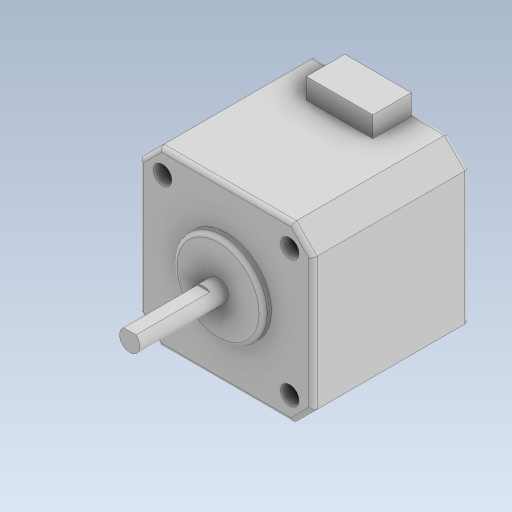
# Autodesk Inventor part: Motor Model
Saved by Autodesk Inventor 2023 (Build 270158000, 158)
## iProperties
Created: 2022-11-09
Part Number: Motor Model
Material: Generic
Document SubType Name: Modeling
Designer: Dave
Density: 1 g/cm^3
Appearance: Default
Author: Dave
Autodesk Inventor part; units mm, degrees
ref_plane "YZ Plane" through (0, 0, 0) normal (1, 0, 0) x (0, 1, 0)
ref_plane "XZ Plane" through (0, 0, 0) normal (0, 1, 0) x (-1, 0, 0)
ref_plane "XY Plane" through (0, 0, 0) normal (0, 0, 1) x (1, 0, 0)
sketch "Sketch1" plane through (0, 0, 0) normal (0, 0, 1) x (1, 0, 0)
  line L0 (5, 0) -> (37.3, 0)
  line L1 (42.3, 5) -> (42.3, 37.3)
  line L2 (37.3, 42.3) -> (5, 42.3)
  line L3 (0, 37.3) -> (0, 5)
  line L4 (5, 42.3) -> (0, 37.3)
  line L5 (42.3, 37.3) -> (37.3, 42.3)
  line L6 (37.3, 0) -> (42.3, 5)
  line L7 (0, 5) -> (5, 0)
  point P0 (0, 0)
  point P1 (42.3, 42.3)
  point P2 (42.3, 0)
  point P3 (0, 42.3)
  dimension "d0" = 42.3
  dimension "d1" = 42.3
  dimension "d2" = 5
  dimension "d3" = 5
  dimension "d4" = 5
  dimension "d5" = 5
  dimension "d6" = 5
  dimension "d7" = 5
  dimension "d8" = 5
  dimension "d9" = 5
  constraints: 16 end point, 8 point on line, 2 parallel, 1 horizontal, 1 perpendicular
  measures "d0" distance of point (0, 42.3) point (42.3, 42.3)
  measures "d1" distance of point (42.3, 42.3) point (42.3, 0)
  measures "d2" distance of L2.end point (0, 42.3)
  measures "d3" distance of L3.start point (0, 42.3)
  measures "d4" distance of L1.end point (42.3, 42.3)
  measures "d5" distance of L2.start point (42.3, 42.3)
  measures "d6" distance of L0.end point (42.3, 0)
  measures "d7" distance of L1.start point (42.3, 0)
  measures "d8" distance of L3.end point (0, 0)
  measures "d9" distance of L0.start point (0, 0)
extrude "Extrusion1" add sketch "Sketch1" along normal blind 38
sketch "Sketch2" plane through (0, 0, 38) normal (0, 0, 1) x (1, 0, 0)
  line L0 (5.65, 36.65) -> (36.65, 36.65) construction
  line L1 (36.65, 36.65) -> (36.65, 5.65) construction
  line L2 (36.65, 5.65) -> (5.65, 5.65) construction
  line L3 (5.65, 5.65) -> (5.65, 36.65) construction
  line L4 (0, 37.3) -> (0, 5) projected
  line L5 (37.3, 42.3) -> (5, 42.3) projected
  circle A0 centre (5.65, 36.65) radius 2.25
  circle A1 centre (36.65, 36.65) radius 2.25
  circle A2 centre (36.65, 5.65) radius 2.25
  circle A3 centre (5.65, 5.65) radius 2.25
  point P0 (0, 0)
  point P1 (5.65, 21.15)
  point P2 (0, 21.15)
  point P3 (21.15, 36.65)
  point P4 (21.15, 42.3)
  dimension "d12" = 31
  dimension "d13" = 4.5
  constraints: 8 end point, 4 centre point, 4 coincident, 4 midpoint, 3 equal length, 3 equal radius, 2 parallel, 1 horizontal, 1 horizontal alignment, 1 perpendicular, 1 vertical alignment
  measures "d12" distance of L0.start L0.end
  measures "d13" diameter of A0
extrude "Extrusion2" cut sketch "Sketch2" against normal blind 10
sketch "Sketch3" plane through (0, 0, 38) normal (0, 0, 1) x (1, 0, 0)
  circle A0 centre (21.15, 21.15) radius 11
  line L0 (37.3, 42.3) -> (5, 42.3) projected
  line L1 (42.3, 5) -> (42.3, 37.3) projected
  point P0 (0, 0)
  point P1 (21.15, 42.3)
  point P2 (42.3, 21.15)
  dimension "d16" = 22
  constraints: 2 midpoint, 1 centre point, 1 horizontal alignment, 1 vertical alignment
  measures "d16" diameter of A0
extrude "Extrusion3" add sketch "Sketch3" along normal blind 2
fillet "Fillet1" radius 1 17 edges at (10.15, 21.15, 40) (21.15, 42.3, 38) (39.8, 39.8, 38) (42.3, 21.15, 38) (39.8, 2.5, 38) (21.15, 0, 38) (2.5, 2.5, 38) (0, 21.15, 38) (2.5, 39.8, 38) (21.15, 42.3, 0) (2.5, 39.8, 0) (39.8, 39.8, 0) (42.3, 21.15, 0) (39.8, 2.5, 0) (21.15, 0, 0) (0, 21.15, 0) (2.5, 2.5, 0)
sketch "Sketch4" plane through (0, 0, 38) normal (0, 0, 1) x (1, 0, 0)
  circle A0 centre (21.15, 21.15) radius 10 projected
  circle A1 centre (21.15, 21.15) radius 2.5
  point P0 (0, 0)
  dimension "d20" = 5
  constraints: 1 centre point, 1 coincident
  measures "d20" diameter of A1
extrude "Extrusion4" add sketch "Sketch4" along normal blind 23.5 contours A1
sketch "Sketch5" plane through (21.15, 21.15, 61.5) normal (0, 0, 1) x (1, 0, 0)
  circle A0 centre (0, 0) radius 2.5 projected
  line L0 (-1.5, 2) -> (1.5, 2)
  circle A1 centre (0, 0) radius 2.5 projected
  point P0 (-21.15, -21.15)
  point P1 (1.5, 2)
  dimension "d23" = 2
  constraints: 2 end point, 1 horizontal, 1 point on circle, 2 other
  measures "d23" distance from line of L0 point (0, 0)
extrude "Extrusion5" cut sketch "Sketch5" against normal blind 18 contours L0 A0 picked at (-0.3466, 2.0912)
sketch "Sketch6" plane through (5, 42.3, 1) normal (0, 1, 0) x (1, 0, 0)
  line L0 (32.3, 0) -> (0, 0) projected
  line L1 (8.05, 0) -> (24.25, 0)
  line L2 (24.25, 0) -> (24.25, -9.4)
  line L3 (24.25, -9.4) -> (8.05, -9.4)
  line L4 (8.05, -9.4) -> (8.05, 0)
  point P0 (-5, 1)
  point P1 (16.15, 0)
  point P2 (24.25, 0)
  dimension "d26" = 16.2
  dimension "d27" = 9.4
  constraints: 8 end point, 2 midpoint, 2 parallel, 1 horizontal, 1 perpendicular, 1 point on line
  measures "d26" distance of L2.end L3.end
  measures "d27" distance of L3.end L1.start
extrude "Extrusion6" add sketch "Sketch6" along normal blind 5
equation "\"d3\" = d2"
equation "\"d4\" = d2"
equation "\"d5\" = d4"
equation "\"d6\" = d2"
equation "\"d7\" = d6"
equation "\"d8\" = d2"
equation "\"d9\" = d8"
body "Solid1"
